Autodesk Inventor part; units mm, degrees
(part 2 of 2)
  spline S109 degree 2 poles (169.673, 4.3946) (169.4639, 4.3946) (169.091, 4.534) (168.9551, 4.6838) knots 0 0 0 1 2 2 2
  spline S110 degree 2 poles (168.9551, 4.6838) (168.8158, 4.8337) (168.6624, 5.2901) (168.6624, 5.6177) knots 0 0 0 1 2 2 2
  line L95 (168.6624, 5.6177) -> (168.6624, 7.7119)
  line L96 (168.6624, 7.7119) -> (169.206, 7.7119)
  line L97 (169.206, 7.7119) -> (169.206, 5.8721)
  spline S111 degree 2 poles (169.206, 5.8721) (169.206, 5.6142) (169.2444, 5.2762) (169.3106, 5.1508) knots 0 0 0 1 2 2 2
  spline S112 degree 2 poles (169.3106, 5.1508) (169.3768, 5.0253) (169.6033, 4.9103) (169.8158, 4.9103) knots 0 0 0 1 2 2 2
  spline S113 degree 2 poles (169.8158, 4.9103) (170.0145, 4.9103) (170.464, 5.1368) (170.6521, 5.3006) knots 0 0 0 1 2 2 2
  line L98 (170.6521, 5.3006) -> (170.6521, 7.7119)
  line L99 (170.6521, 7.7119) -> (171.1957, 7.7119)
  line L100 (171.1957, 7.7119) -> (171.1957, 4.4852)
  spline S114 degree 2 poles (175.5515, 4.4085) (175.1333, 4.4085) (174.426, 4.6908) (174.1681, 4.973) knots 0 0 0 1 2 2 2
  spline S115 degree 2 poles (174.1681, 4.973) (173.9102, 5.2518) (173.628, 6.0881) (173.628, 6.6317) knots 0 0 0 1 2 2 2
  spline S116 degree 2 poles (173.628, 6.6317) (173.628, 7.1718) (173.9033, 7.9733) (174.1646, 8.2695) knots 0 0 0 1 2 2 2
  spline S117 degree 2 poles (174.1646, 8.2695) (174.4225, 8.5587) (175.1264, 8.8619) (175.5619, 8.8619) knots 0 0 0 1 2 2 2
  spline S118 degree 2 poles (175.5619, 8.8619) (175.778, 8.8619) (176.1578, 8.7991) (176.3181, 8.7504) knots 0 0 0 1 2 2 2
  spline S119 degree 2 poles (176.3181, 8.7504) (176.4575, 8.7051) (176.7467, 8.5761) (176.8896, 8.4995) knots 0 0 0 1 2 2 2
  line L101 (176.8896, 8.4995) -> (176.8896, 7.8095)
  line L102 (176.8896, 7.8095) -> (176.8443, 7.8095)
  spline S120 degree 2 poles (176.8443, 7.8095) (176.7676, 7.8792) (176.5307, 8.0743) (176.3599, 8.1684) knots 0 0 0 1 2 2 2
  spline S121 degree 2 poles (176.3599, 8.1684) (176.1961, 8.259) (175.8094, 8.374) (175.5585, 8.374) knots 0 0 0 1 2 2 2
  spline S122 degree 2 poles (175.5585, 8.374) (175.2832, 8.374) (174.7919, 8.1475) (174.6072, 7.9315) knots 0 0 0 1 2 2 2
  spline S123 degree 2 poles (174.6072, 7.9315) (174.426, 7.7119) (174.2239, 7.0464) (174.2239, 6.6317) knots 0 0 0 1 2 2 2
  spline S124 degree 2 poles (174.2239, 6.6317) (174.2239, 6.1892) (174.4364, 5.5515) (174.6211, 5.332) knots 0 0 0 1 2 2 2
  spline S125 degree 2 poles (174.6211, 5.332) (174.8023, 5.1194) (175.2867, 4.9034) (175.5585, 4.9034) knots 0 0 0 1 2 2 2
  spline S126 degree 2 poles (175.5585, 4.9034) (175.8059, 4.9034) (176.2275, 5.0253) (176.3913, 5.1159) knots 0 0 0 1 2 2 2
  spline S127 degree 2 poles (176.3913, 5.1159) (176.5481, 5.2065) (176.7816, 5.3947) (176.8478, 5.4609) knots 0 0 0 1 2 2 2
  line L103 (176.8478, 5.4609) -> (176.8896, 5.4609)
  line L104 (176.8896, 5.4609) -> (176.8896, 4.7779)
  spline S128 degree 2 poles (176.8896, 4.7779) (176.7467, 4.7117) (176.4958, 4.5897) (176.3181, 4.534) knots 0 0 0 1 2 2 2
  spline S129 degree 2 poles (176.3181, 4.534) (176.1299, 4.4713) (175.8094, 4.4085) (175.5515, 4.4085) knots 0 0 0 1 2 2 2
  point P0 (0, 0)
  constraints: 2 other
extrude "Extrusión8" cut sketch "Boceto10" against normal blind 0.3
sketch "Boceto11" plane through (0, 0, 0) normal (0, -1, 0) x (1, 0, 0)
  line L0 (10.005, -7.4262) -> (-19.8869, -7.4262) construction
  line L1 (-19.8869, -7.4262) -> (-19.8869, 2.4029) construction
  line L2 (-19.8869, 2.4029) -> (10.005, 2.4029) construction
  line L3 (10.005, 2.4029) -> (10.005, -7.4262) construction
  line L4 (7.6083, -4.8816) -> (7.9406, -4.8816)
  line L5 (7.9406, -4.8816) -> (7.9406, -7.0351)
  line L6 (7.9406, -7.0351) -> (8.5929, -5.5704)
  line L7 (8.5929, -5.5704) -> (8.7955, -5.5704)
  line L8 (8.7955, -5.5704) -> (9.4418, -7.0351)
  line L9 (9.4418, -7.0351) -> (9.4418, -4.8816)
  line L10 (9.4418, -4.8816) -> (9.7518, -4.8816)
  line L11 (9.7518, -4.8816) -> (9.7518, -7.3816)
  line L12 (9.7518, -7.3816) -> (9.298, -7.3816)
  line L13 (9.298, -7.3816) -> (8.674, -5.9898)
  line L14 (8.674, -5.9898) -> (8.0703, -7.3816)
  line L15 (8.0703, -7.3816) -> (7.6083, -7.3816)
  line L16 (7.6083, -7.3816) -> (7.6083, -4.8816)
  line L17 (6.5184, -4.8816) -> (6.5184, -7.0858)
  line L18 (6.5184, -7.0858) -> (7.3571, -7.0858)
  line L19 (7.3571, -7.0858) -> (7.3571, -7.3816)
  line L20 (7.3571, -7.3816) -> (5.3474, -7.3816)
  line L21 (5.3474, -7.3816) -> (5.3474, -7.0858)
  line L22 (5.3474, -7.0858) -> (6.1861, -7.0858)
  line L23 (6.1861, -7.0858) -> (6.1861, -4.8816)
  line L24 (6.1861, -4.8816) -> (6.5184, -4.8816)
  spline S0 degree 2 poles (4.1177, -4.837) (4.3608, -4.837) (4.772, -5.0011) (4.922, -5.1652) knots 0 0 0 1 2 2 2
  spline S1 degree 2 poles (4.922, -5.1652) (5.0719, -5.3273) (5.236, -5.8135) (5.236, -6.1296) knots 0 0 0 1 2 2 2
  spline S2 degree 2 poles (5.236, -6.1296) (5.236, -6.4436) (5.0759, -6.9095) (4.924, -7.0817) knots 0 0 0 1 2 2 2
  spline S3 degree 2 poles (4.924, -7.0817) (4.7741, -7.2499) (4.3648, -7.4262) (4.1116, -7.4262) knots 0 0 0 1 2 2 2
  spline S4 degree 2 poles (4.1116, -7.4262) (3.986, -7.4262) (3.7652, -7.3897) (3.672, -7.3613) knots 0 0 0 1 2 2 2
  spline S5 degree 2 poles (3.672, -7.3613) (3.5909, -7.335) (3.4228, -7.26) (3.3397, -7.2155) knots 0 0 0 1 2 2 2
  line L25 (3.3397, -7.2155) -> (3.3397, -6.8143)
  line L26 (3.3397, -6.8143) -> (3.366, -6.8143)
  spline S6 degree 2 poles (3.366, -6.8143) (3.4106, -6.8548) (3.5484, -6.9683) (3.6476, -7.023) knots 0 0 0 1 2 2 2
  spline S7 degree 2 poles (3.6476, -7.023) (3.7429, -7.0757) (3.9677, -7.1425) (4.1136, -7.1425) knots 0 0 0 1 2 2 2
  spline S8 degree 2 poles (4.1136, -7.1425) (4.2737, -7.1425) (4.5593, -7.0108) (4.6667, -6.8852) knots 0 0 0 1 2 2 2
  spline S9 degree 2 poles (4.6667, -6.8852) (4.772, -6.7576) (4.8895, -6.3706) (4.8895, -6.1296) knots 0 0 0 1 2 2 2
  spline S10 degree 2 poles (4.8895, -6.1296) (4.8895, -5.8723) (4.766, -5.5015) (4.6586, -5.3739) knots 0 0 0 1 2 2 2
  spline S11 degree 2 poles (4.6586, -5.3739) (4.5532, -5.2503) (4.2716, -5.1247) (4.1136, -5.1247) knots 0 0 0 1 2 2 2
  spline S12 degree 2 poles (4.1136, -5.1247) (3.9698, -5.1247) (3.7246, -5.1956) (3.6294, -5.2483) knots 0 0 0 1 2 2 2
  spline S13 degree 2 poles (3.6294, -5.2483) (3.5382, -5.3009) (3.4025, -5.4103) (3.364, -5.4488) knots 0 0 0 1 2 2 2
  line L27 (3.364, -5.4488) -> (3.3397, -5.4488)
  line L28 (3.3397, -5.4488) -> (3.3397, -5.0518)
  spline S14 degree 2 poles (3.3397, -5.0518) (3.4228, -5.0133) (3.5686, -4.9424) (3.672, -4.9099) knots 0 0 0 1 2 2 2
  spline S15 degree 2 poles (3.672, -4.9099) (3.7814, -4.8735) (3.9677, -4.837) (4.1177, -4.837) knots 0 0 0 1 2 2 2
  point P0 (0, 0)
  constraints: 2 other
extrude "Extrusión9" cut sketch "Boceto11" against normal blind 0.3
sketch "Boceto12" plane through (0, 2, 0) normal (0, 1, 0) x (1, 0, 0)
  line L0 (89.4618, 42) -> (98.4618, 42) projected
  line L1 (0, 47.5) -> (0, 48)
  line L2 (0, 100) -> (0, 0) projected
  line L3 (0, 47.5) -> (0, 47)
  line L4 (0, 47) -> (180, 47)
  line L5 (0, 48) -> (180, 48)
  line L6 (180, 47) -> (180, 48)
  constraints: 10 end point, 2 point on line
extrude "Extrusión11" cut sketch "Boceto12" against normal blind 0.3
extrude "Extrusión12" cut sketch "Boceto2" against normal blind 19.8 contours A0 | A1 | L13 L12 L11 L10 L9 | L14 L15 L16 L17 L18 | L19 L20 L21 L22 L23 | L24 L25 L26 L27 | A2 | A3
